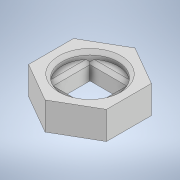
# Autodesk Inventor part: inserttest
Saved by Autodesk Inventor 2022 (Build 260153000, 153)
## iProperties
Created: 2022-03-19
Part Number: inserttest
Material: Generic
Document SubType Name: Modeling
Designer: zac-h
Density: 1 g/cm^3
Appearance: Default
Author: zac-h
Autodesk Inventor part; units mm, degrees
ref_plane "YZ Plane" through (0, 0, 0) normal (1, 0, 0) x (0, 1, 0)
ref_plane "XZ Plane" through (0, 0, 0) normal (0, 1, 0) x (-1, 0, 0)
ref_plane "XY Plane" through (0, 0, 0) normal (0, 0, 1) x (1, 0, 0)
sketch "Sketch1" plane through (0, 0, 0) normal (0, 1, 0) x (-1, 0, 0)
  line L0 (0, -8.0829) -> (-7, -4.0415)
  line L1 (-7, -4.0415) -> (-7, 4.0415)
  line L2 (-7, 4.0415) -> (0, 8.0829)
  line L3 (0, 8.0829) -> (7, 4.0415)
  line L4 (7, 4.0415) -> (7, -4.0415)
  line L5 (7, -4.0415) -> (0, -8.0829)
  line L6 (-3.315, 3.315) -> (3.315, 3.315)
  line L7 (3.315, 3.315) -> (3.315, -3.315)
  line L8 (3.315, -3.315) -> (-3.315, -3.315)
  line L9 (-3.315, -3.315) -> (-3.315, 3.315)
  line L10 (-3.315, 3.315) -> (3.315, -3.315) construction
  line L11 (3.315, 3.315) -> (-3.315, -3.315) construction
  point P0 (0, 0)
  point P1 (0, 0)
  dimension "d0" = 14
  dimension "d1" = 6.63
  constraints: 24 end point, 2 midpoint, 2 parallel, 2 perpendicular, 1 coincident, 1 horizontal, 1 vertical, 13 other
  measures "d0" distance between parallel lines of L1 L4
  measures "d1" distance of L8.end L6.start
extrude "Extrusion1" add sketch "Sketch1" along normal blind 5
sketch "Sketch2" plane through (0, 5, 0) normal (0, 1, 0) x (1, 0, 0)
  circle A0 centre (0, 0) radius 5.025
  dimension "d4" = 10.05
  constraints: 1 centre point, 1 coincident
  measures "d4" diameter of A0
extrude "Extrusion2" cut sketch "Sketch2" against normal blind 1.27
chamfer "Chamfer1" distance 0.6 angle 45 5 edges at (-3.315, 3.73, 0) (0, 3.73, 3.315) (3.315, 3.73, 0) (0, 3.73, -3.315) (-5.025, 5, 0)
chamfer "Chamfer2" distance 0.6 angle 45 4 edges at (-3.315, 0, 0) (0, 0, 3.315) (3.315, 0, 0) (0, 0, -3.315)
body "Solid1"
